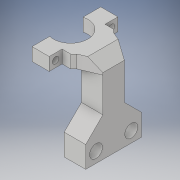
# Autodesk Inventor part: КВ33.044.207 - Крепление вакумной присоски
Saved by Autodesk Inventor 2019 (Build 230136000, 136)
## iProperties
Created: 2019-08-29
Part Number: КВ33.044.207 - Крепление вакумной присоски
Material: Типовые
Document SubType Name: Modeling
Designer: Петров Иван
Density: 1 g/cm^3
Appearance: По умолчанию
Mass: 0.831375 g
Surface Area: 8.87885 cm^2
Volume: 0.831375 cm^3
Author: Петров Иван
Autodesk Inventor part; units mm, degrees
ref_plane "YZ Plane" through (0, 0, 0) normal (1, 0, 0) x (0, 1, 0)
ref_plane "XZ Plane" through (0, 0, 0) normal (0, 1, 0) x (-1, 0, 0)
sketch "Эскиз1" plane through (0, 0, 0) normal (1, 0, 0) x (0, 1, 0)
  line L0 (0, 0) -> (0, -8.197)
  circle A0 centre (0, 0) radius 1.5
  circle A1 centre (0, -8.197) radius 1.5
  line L1 (-2.5, 2.4015) -> (2.5, 2.4015)
  line L2 (2.5, 2.4015) -> (2.5, -10.5985)
  line L3 (2.5, -10.5985) -> (-2.5, -10.5985)
  line L4 (-2.5, -10.5985) -> (-2.5, 2.4015)
  line L5 (-2.5, 2.4015) -> (2.5, -10.5985) construction
  line L6 (2.5, 2.4015) -> (-2.5, -10.5985) construction
  point P0 (0, -4.0985)
  dimension "d0" = 8.197
  dimension "d1" = 3
  dimension "d2" = 3
  dimension "d3" = 5
  dimension "d4" = 13
  constraints: 14 end point, 3 midpoint, 2 centre point, 2 coincident, 2 parallel, 1 horizontal, 1 perpendicular, 1 vertical
  measures "d0" distance of L0.start L0.end
  measures "d1" diameter of A0
  measures "d2" diameter of A1
  measures "d3" distance of L2.end L3.end
  measures "d4" distance of L1.end L2.end
extrude "Выдавливание1" add sketch "Эскиз1" along normal blind 5
sketch "Эскиз2" plane through (0, 2.5, 2.4015) normal (0, 1, 0) x (1, 0, 0)
  line L0 (0, 0) -> (5, 0) projected
  line L1 (2.5, 0) -> (2.5, 13)
  line L2 (0, 13) -> (5, 13) projected
  line L3 (0, 13) -> (0, 0) projected
  line L4 (5, 4) -> (0, 4)
  line L5 (0, 4) -> (0, 9)
  line L6 (0, 9) -> (5, 9)
  line L7 (5, 9) -> (5, 4)
  line L8 (5, 4) -> (0, 9) construction
  line L9 (0, 4) -> (5, 9) construction
  point P0 (0, 2.4015)
  point P1 (2.5, 6.5)
  dimension "d7" = 5
  constraints: 14 end point, 5 midpoint, 2 parallel, 1 horizontal, 1 perpendicular, 1 point on line
  measures "d7" distance of L4.end L5.end
extrude "Выдавливание2" add sketch "Эскиз2" along normal blind 15 contours L3 L6 L1 L4 | L1 L6 L7 L4
sketch "Эскиз3" plane through (0, 0, 0) normal (-1, 0, 0) x (0, 0, 1)
  line L0 (-1.5985, 17.5) -> (-6.5985, 17.5) projected
  line L1 (-4.0985, 17.5) -> (-4.0985, 16)
  line L2 (-9.0985, 14.5) -> (0.9015, 14.5)
  line L3 (0.9015, 14.5) -> (0.9015, 17.5)
  line L4 (0.9015, 17.5) -> (-9.0985, 17.5)
  line L5 (-9.0985, 17.5) -> (-9.0985, 14.5)
  line L6 (-9.0985, 14.5) -> (0.9015, 17.5) construction
  line L7 (0.9015, 14.5) -> (-9.0985, 17.5) construction
  point P0 (0, 0)
  dimension "d10" = 1.5
  dimension "d11" = 10
  dimension "d12" = 3
  constraints: 14 end point, 3 midpoint, 2 parallel, 1 horizontal, 1 perpendicular, 1 vertical
  measures "d10" distance of L1.start L1.end
  measures "d11" distance of L4.end L3.end
  measures "d12" distance of L3.end L2.end
extrude "Выдавливание3" add sketch "Эскиз3" along normal blind 10
sketch "Эскиз4" plane through (0, 17.5, 2.4015) normal (0, 1, 0) x (1, 0, 0)
  line L0 (0, 1.5) -> (-10, 1.5) projected
  line L1 (-5, 1.5) -> (-5, 11.5)
  line L2 (0, 11.5) -> (-10, 11.5) projected
  circle A0 centre (-5, 6.5) radius 4
  line L3 (-10, 1.5) -> (-10, 11.5) projected
  line L4 (-10, 1.5) -> (-10, 11.5)
  point P0 (0, 2.4015)
  point P1 (-7.0808, 9.9162)
  point P2 (-7.0808, 3.0838)
  dimension "d15" = 8
  constraints: 4 end point, 3 midpoint, 2 point on circle, 1 centre point, 1 collinear
  measures "d15" diameter of A0
extrude "Выдавливание4" cut sketch "Эскиз4" against normal blind 10 contours A0 L1 | L1 A0
chamfer "Фаска1" distance 2.5 angle 45 2 edges at (0, 16, -1.5985) (0, 16, -6.5985)
chamfer "Фаска2" distance 4 angle 45 2 edges at (2.5, 2.5, -6.5985) (2.5, 2.5, -1.5985)
sketch "Эскиз5" plane through (-10, 0, 0) normal (-1, 0, 0) x (0, 0, 1)
  line L0 (-9.0985, 14.5) -> (0.9015, 14.5) projected
  line L1 (-9.0985, 14.5) -> (-12.0985, 14.5)
  line L2 (0.9015, 17.5) -> (-9.0985, 17.5) projected
  line L3 (-12.0985, 14.5) -> (-9.0985, 14.5)
  line L4 (-9.0985, 14.5) -> (-9.0985, 17.5)
  line L5 (-9.0985, 17.5) -> (-12.0985, 17.5)
  line L6 (-12.0985, 17.5) -> (-12.0985, 14.5)
  line L7 (0.9015, 17.5) -> (3.9015, 17.5)
  line L8 (3.9015, 17.5) -> (3.9015, 14.5)
  line L9 (3.9015, 14.5) -> (0.9015, 14.5)
  line L10 (0.9015, 14.5) -> (0.9015, 17.5)
  line L11 (-9.0985, 17.5) -> (0.9015, 17.5)
  line L12 (0.9015, 17.5) -> (0.9015, 14.5)
  line L13 (0.9015, 14.5) -> (-9.0985, 14.5)
  line L14 (-9.0985, 14.5) -> (-9.0985, 17.5)
  point P0 (0, 0)
  dimension "d24" = 3
  dimension "d25" = 3
  dimension "d26" = 3
  constraints: 26 end point, 6 parallel, 4 horizontal, 3 perpendicular
  measures "d24" distance of L0.start L1.end
  measures "d25" distance of L8.end L9.end
  measures "d26" distance of L7.end L8.end
extrude "Выдавливание5" cut sketch "Эскиз5" against normal blind 4
sketch "Эскиз6" plane through (-6, 0, 0) normal (-1, 0, 0) x (0, 0, 1)
  line L0 (-9.0985, 17.5) -> (-9.0985, 14.5) projected
  line L1 (-9.0985, 17.5) -> (-12.0985, 17.5)
  line L2 (-12.0985, 17.5) -> (-12.0985, 14.5)
  line L3 (-12.0985, 14.5) -> (-9.0985, 14.5)
  line L4 (-9.0985, 14.5) -> (-9.0985, 17.5)
  line L5 (-1.5985, 14.5) -> (-6.5985, 14.5) projected
  line L6 (-4.0985, 14.5) -> (-4.0985, 15.1912)
  line L7 (-12.0985, 17.5) -> (-10.5985, 17.5)
  line L8 (-12.0985, 16) -> (-12.0985, 17.5)
  circle A0 centre (-10.5985, 16) radius 0.75
  point P0 (0, 0)
  dimension "d29" = 3
  dimension "d30" = 3
  dimension "d33" = 1.5
  constraints: 14 end point, 2 horizontal, 2 parallel, 1 centre point, 1 midpoint, 1 perpendicular, 1 vertical
  measures "d29" distance of L3.end L2.end
  measures "d30" distance of L2.end L1.end
  measures "d33" diameter of A0
ref_plane "РабПлоскость1" through (-1, 17.5, -4.0985) normal (0, 0, -1) x (-1, 0, 0)
extrude "Выдавливание6" add sketch "Эскиз6" against normal blind 4
mirror "Зеркальное отражение1" about plane through (-1, 17.5, -4.0985) normal (0, 0, -1) of "Выдавливание6"
sketch "Эскиз7" plane through (-6, 0, 0) normal (-1, 0, 0) x (0, 0, 1)
  line L0 (-7.9715, 17.5) -> (-12.0985, 17.5) projected
  circle A0 centre (-10.5985, 16) radius 0.75 projected
  line L1 (-7.9715, 14.5) -> (-12.0985, 14.5) projected
  line L2 (-7.9715, 17.5) -> (-7.9715, 14.5) projected
  line L3 (-7.9715, 17.5) -> (-12.0985, 17.5) projected
  line L4 (-12.0985, 17.5) -> (-12.0985, 14.5) projected
  circle A1 centre (2.4015, 16) radius 0.75 projected
  line L5 (-0.2255, 14.5) -> (-0.2255, 17.5) projected
  line L6 (3.9015, 14.5) -> (-0.2255, 14.5) projected
  line L7 (3.9015, 17.5) -> (3.9015, 14.5) projected
  line L8 (-0.2255, 17.5) -> (3.9015, 17.5) projected
  line L9 (-7.9715, 17.5) -> (-7.9715, 14.5) projected
  line L10 (-0.2255, 14.5) -> (-7.9715, 14.5) projected
  line L11 (-0.2255, 14.5) -> (-0.2255, 17.5) projected
  line L12 (-7.9715, 17.5) -> (-0.2255, 17.5) projected
  point P0 (0, 0)
chamfer "Фаска3" distance 2.5 angle 45 3 edges at (2.4995, 16, -1.5985) (2.4995, 16, -6.5985) (5, 17.5, -4.0985)
